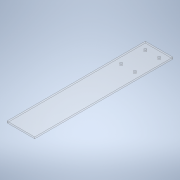
# Autodesk Inventor part: 10x2 Lexan
Saved by Autodesk Inventor 2021 (Build 250183000, 183)
## iProperties
Created: 2020-01-14
Part Number: 10x2 Lexan
Material: Polycarbonate, Clear
Document SubType Name: Modeling
Designer: aidan
Density: 1.2 g/cm^3
Appearance: Polycarbonate - Clear
Author: aidan
Autodesk Inventor part; units mm, degrees
ref_plane "YZ Plane" through (0, 0, 0) normal (1, 0, 0) x (0, 1, 0)
ref_plane "XZ Plane" through (0, 0, 0) normal (0, 1, 0) x (-1, 0, 0)
ref_plane "XY Plane" through (0, 0, 0) normal (0, 0, 1) x (1, 0, 0)
sketch "Sketch1" plane through (0, 0, 0) normal (0, 1, 0) x (-1, 0, 0)
  line L0 (374.9202, -9.4574) -> (324.1202, -9.4574)
  line L1 (324.1202, -9.4574) -> (324.1202, -263.4574)
  line L2 (324.1202, -263.4574) -> (374.9202, -263.4574)
  line L3 (374.9202, -263.4574) -> (374.9202, -9.4574)
  point P0 (0, 0)
  dimension "d0" = 254
  dimension "d1" = 50.8
  constraints: 8 end point, 2 parallel, 1 horizontal, 1 perpendicular
  measures "d0" distance of L2.end L0.start
  measures "d1" distance of L1.end L2.end
extrude "Extrusion1" add sketch "Sketch1" along normal blind 2.9972
sketch "Sketch2" plane through (0, 2.9972, 0) normal (0, 1, 0) x (1, 0, 0)
  line L0 (-336.8202, 206.3074) -> (-362.2202, 206.3074) construction
  line L1 (-362.2202, 206.3074) -> (-362.2202, 250.7574) construction
  line L2 (-362.2202, 250.7574) -> (-336.8202, 250.7574) construction
  line L3 (-336.8202, 250.7574) -> (-336.8202, 206.3074) construction
  line L4 (-336.8202, 206.3074) -> (-362.2202, 250.7574) construction
  line L5 (-362.2202, 206.3074) -> (-336.8202, 250.7574) construction
  line L6 (-324.1202, 263.4574) -> (-374.9202, 263.4574) projected
  line L7 (-349.5202, 228.5324) -> (-349.5202, 263.4574) construction
  circle A0 centre (-362.2202, 250.7574) radius 2.1828
  circle A1 centre (-336.8202, 250.7574) radius 2.1828
  circle A2 centre (-336.8202, 206.3074) radius 2.1828
  circle A3 centre (-362.2202, 206.3074) radius 2.1828
  point P0 (0, 0)
  dimension "d4" = 25.4
  dimension "d5" = 44.45
  dimension "d6" = 12.7
  dimension "d7" = 4.3656
  constraints: 14 end point, 4 centre point, 4 coincident, 3 equal radius, 3 midpoint, 2 parallel, 1 horizontal, 1 perpendicular, 1 vertical
  measures "d4" distance of L1.end L2.end
  measures "d5" distance of L2.end L0.start
  measures "d6" distance between parallel lines of L2 L6
  measures "d7" diameter of A0
extrude "Extrusion2" cut sketch "Sketch2" against normal through all
body "Solid1"
